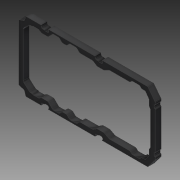
# Autodesk Inventor part: A0008269480
Saved by Autodesk Inventor 2014 SP2 (Build 180246200, 246)
## iProperties
Created: 2014-09-20
Part Number: A0008269480
Material: Rubber
Document SubType Name: Modeling
Designer: Lukasz Szmit
Density: 0.93 g/cm^3
Appearance: Rubber - Black - Version 1.1
Author: Lukasz Szmit
Autodesk Inventor part; units mm, degrees
ref_plane "YZ Plane" through (0, 0, 0) normal (1, 0, 0) x (0, 1, 0)
ref_plane "XZ Plane" through (0, 0, 0) normal (0, 1, 0) x (-1, 0, 0)
ref_plane "XY Plane" through (0, 0, 0) normal (0, 0, 1) x (1, 0, 0)
sketch "Sketch1" plane through (0, 0, 0) normal (0, 1, 0) x (-1, 0, 0)
  line L0 (206.8069, 83.1723) -> (206.8069, -83.1723)
  line L1 (193.4069, -67.3858) -> (193.4069, 67.3858)
  line L2 (-189.8501, 49.189) -> (-189.8501, -94.3805)
  line L3 (-189.4414, -50.7006) -> (-186.55, -55.6572)
  line L4 (-186.1413, -57.1689) -> (-186.1413, -72.6556)
  line L5 (-185.5922, -74.3857) -> (-175.4668, -88.73)
  line L6 (-200.9413, -60) -> (-200.9413, -64.9002)
  line L7 (-204.4413, -74.3803) -> (-204.4413, -69.2877)
  line L8 (-204.4501, -55.6105) -> (-204.4501, 55.6105)
  arc A0 (-203.2747, -67.8252) -> (-200.9413, -64.9002) centre (-203.9413, -64.9002) ccw
  arc A1 (-200.9413, -60) -> (-203.2805, -57.0737) centre (-203.9413, -60) ccw
  line L9 (-203.8197, -76.2088) -> (-182.8943, -103.4284)
  arc A2 (-182.8943, -103.4284) -> (-180.5159, -104.6) centre (-180.5159, -101.6) ccw
  arc A3 (-175.4668, -88.73) -> (-173.0159, -90) centre (-173.0159, -87) ccw
  arc A4 (-204.4413, -74.3803) -> (-203.8197, -76.2088) centre (-201.4413, -74.3803) ccw
  arc A5 (-186.1413, -72.6556) -> (-185.5922, -74.3857) centre (-183.1413, -72.6556) ccw
  arc A6 (-186.1413, -57.1689) -> (-186.55, -55.6572) centre (-189.1413, -57.1689) ccw
  arc A7 (-189.8501, -49.189) -> (-189.4414, -50.7006) centre (-186.8501, -49.189) ccw
  arc A8 (-204.4501, -55.6105) -> (-203.2805, -57.0737) centre (-202.9501, -55.6105) ccw
  arc A9 (-203.2747, -67.8252) -> (-204.4413, -69.2877) centre (-202.9413, -69.2877) ccw
  line L10 (-155.0159, -96.0718) -> (-137.0159, -96.0718)
  line L11 (-173.0159, -90) -> (-166.0159, -90)
  arc A10 (-126.0159, -90) -> (-131.5159, -93.0359) centre (-126.0159, -96.5) ccw
  arc A11 (-137.0159, -96.0718) -> (-131.5159, -93.0359) centre (-137.0159, -89.5718) ccw
  arc A12 (-160.5159, -93.0359) -> (-155.0159, -96.0718) centre (-155.0159, -89.5718) ccw
  arc A13 (-160.5159, -93.0359) -> (-166.0159, -90) centre (-166.0159, -96.5) ccw
  line L12 (-64.4945, -89.2551) -> (-51.3322, -82.3449)
  line L13 (-126.0159, -90) -> (-67.5159, -90)
  line L14 (-48.3108, -81.6) -> (-31.3108, -81.6)
  line L15 (-17.9251, -88.9697) -> (-27.7991, -82.6303)
  arc A14 (-67.5159, -90) -> (-64.4945, -89.2551) centre (-67.5159, -83.5) ccw
  arc A15 (-48.3108, -81.6) -> (-51.3322, -82.3449) centre (-48.3108, -88.1) ccw
  arc A16 (-17.9251, -88.9697) -> (-14.4134, -90) centre (-14.4134, -83.5) ccw
  arc A17 (-27.7991, -82.6303) -> (-31.3108, -81.6) centre (-31.3108, -88.1) ccw
  line L16 (-14.4134, -90) -> (20.5866, -90)
  line L17 (50.4322, -99.4607) -> (35.4322, -99.4607)
  line L18 (25.1828, -91.9038) -> (30.836, -97.5569)
  line L19 (60.6815, -91.9038) -> (55.0284, -97.5569)
  line L20 (65.2777, -90) -> (73.2777, -90)
  line L21 (77.8739, -91.9038) -> (83.527, -97.5569)
  arc A18 (25.1828, -91.9038) -> (20.5866, -90) centre (20.5866, -96.5) ccw
  arc A19 (50.4322, -99.4607) -> (55.0284, -97.5569) centre (50.4322, -92.9607) ccw
  arc A20 (65.2777, -90) -> (60.6815, -91.9038) centre (65.2777, -96.5) ccw
  arc A21 (77.8739, -91.9038) -> (73.2777, -90) centre (73.2777, -96.5) ccw
  arc A22 (30.836, -97.5569) -> (35.4322, -99.4607) centre (35.4322, -92.9607) ccw
  line L22 (88.1232, -99.4607) -> (101.1232, -99.4607)
  arc A23 (83.527, -97.5569) -> (88.1232, -99.4607) centre (88.1232, -92.9607) ccw
  line L23 (105.7194, -97.5569) -> (116.7725, -86.5038)
  arc A24 (101.1232, -99.4607) -> (105.7194, -97.5569) centre (101.1232, -92.9607) ccw
  line L24 (121.3687, -84.6) -> (136.3687, -84.6)
  line L25 (139.6187, -85.4708) -> (145.9551, -89.1292)
  arc A25 (121.3687, -84.6) -> (116.7725, -86.5038) centre (121.3687, -91.1) ccw
  arc A26 (139.6187, -85.4708) -> (136.3687, -84.6) centre (136.3687, -91.1) ccw
  arc A27 (145.9551, -89.1292) -> (149.2051, -90) centre (149.2051, -83.5) ccw
  line L26 (149.2051, -90) -> (163.3581, -90)
  line L27 (165.0901, -89) -> (164.9354, -89.2679)
  line L28 (166.4987, -88.2751) -> (171.369, -87.8626)
  line L29 (175.0876, -86.2889) -> (191.1741, -72.2889)
  arc A28 (163.3581, -90) -> (165.0901, -89) centre (163.3581, -88) ccw
  arc A29 (166.4987, -88.2751) -> (164.9354, -89.2679) centre (166.6675, -90.2679) ccw
  arc A30 (171.369, -87.8626) -> (175.0876, -86.2889) centre (170.8204, -81.3858) ccw
  arc A31 (191.1741, -72.2889) -> (193.4069, -67.3858) centre (186.9069, -67.3858) ccw
  line L30 (188.8967, -93.6379) -> (186.5552, -102.3765)
  line L31 (193.4929, -89.0417) -> (204.5834, -86.07)
  arc A32 (193.4929, -89.0417) -> (188.8967, -93.6379) centre (195.1753, -95.3202) ccw
  arc A33 (204.5834, -86.07) -> (206.8069, -83.1723) centre (203.8069, -83.1723) ccw
  arc A34 (183.6575, -104.6) -> (186.5552, -102.3765) centre (183.6575, -101.6) ccw
  line L32 (-41.4608, -99.75) -> (-36.5608, -99.75) construction
  line L33 (-36.5608, -94.9) -> (-41.4608, -94.9)
  arc A35 (-41.4608, -94.9) -> (-44.2842, -103.6935) centre (-41.4608, -99.75) ccw
  arc A36 (-32.7112, -96.8) -> (-36.5608, -94.9) centre (-36.5608, -99.75) ccw
  line L34 (-32.7112, -96.8) -> (-27.8608, -96.8)
  arc A37 (-23.0293, -101.2273) -> (-27.8608, -96.8) centre (-27.8608, -101.65) ccw
  line L35 (-44.5753, -104.6) -> (-180.5159, -104.6)
  line L36 (-22.7342, -104.6) -> (-23.0293, -101.2273)
  arc A38 (-44.5753, -104.6) -> (-44.2842, -103.6935) centre (-44.5753, -104.1) ccw
  line L37 (183.6575, -104.6) -> (139.6187, -104.6)
  line L38 (117.7776, -104.6) -> (-22.7342, -104.6)
  line L39 (-189.4414, 50.7006) -> (-186.55, 55.6572)
  line L40 (-186.1413, 57.1689) -> (-186.1413, 72.6556)
  line L41 (-185.5922, 74.3857) -> (-175.4668, 88.73)
  line L42 (-200.9413, 60) -> (-200.9413, 64.9002)
  line L43 (-204.4413, 74.3803) -> (-204.4413, 69.2877)
  arc A39 (-200.9413, 64.9002) -> (-203.2747, 67.8252) centre (-203.9413, 64.9002) ccw
  arc A40 (-203.2805, 57.0737) -> (-200.9413, 60) centre (-203.9413, 60) ccw
  line L44 (-203.8197, 76.2088) -> (-182.8943, 103.4284)
  arc A41 (-180.5159, 104.6) -> (-182.8943, 103.4284) centre (-180.5159, 101.6) ccw
  arc A42 (-173.0159, 90) -> (-175.4668, 88.73) centre (-173.0159, 87) ccw
  arc A43 (-203.8197, 76.2088) -> (-204.4413, 74.3803) centre (-201.4413, 74.3803) ccw
  arc A44 (-185.5922, 74.3857) -> (-186.1413, 72.6556) centre (-183.1413, 72.6556) ccw
  arc A45 (-186.55, 55.6572) -> (-186.1413, 57.1689) centre (-189.1413, 57.1689) ccw
  arc A46 (-189.4414, 50.7006) -> (-189.8501, 49.189) centre (-186.8501, 49.189) ccw
  arc A47 (-203.2805, 57.0737) -> (-204.4501, 55.6105) centre (-202.9501, 55.6105) ccw
  arc A48 (-204.4413, 69.2877) -> (-203.2747, 67.8252) centre (-202.9413, 69.2877) ccw
  line L45 (-155.0159, 96.0718) -> (-137.0159, 96.0718)
  line L46 (-173.0159, 90) -> (-166.0159, 90)
  arc A49 (-131.5159, 93.0359) -> (-126.0159, 90) centre (-126.0159, 96.5) ccw
  arc A50 (-131.5159, 93.0359) -> (-137.0159, 96.0718) centre (-137.0159, 89.5718) ccw
  arc A51 (-155.0159, 96.0718) -> (-160.5159, 93.0359) centre (-155.0159, 89.5718) ccw
  arc A52 (-166.0159, 90) -> (-160.5159, 93.0359) centre (-166.0159, 96.5) ccw
  line L47 (-64.4945, 89.2551) -> (-51.3322, 82.3449)
  line L48 (-126.0159, 90) -> (-67.5159, 90)
  line L49 (-48.3108, 81.6) -> (-31.3108, 81.6)
  line L50 (-17.9251, 88.9697) -> (-27.7991, 82.6303)
  arc A53 (-64.4945, 89.2551) -> (-67.5159, 90) centre (-67.5159, 83.5) ccw
  arc A54 (-51.3322, 82.3449) -> (-48.3108, 81.6) centre (-48.3108, 88.1) ccw
  arc A55 (-14.4134, 90) -> (-17.9251, 88.9697) centre (-14.4134, 83.5) ccw
  arc A56 (-31.3108, 81.6) -> (-27.7991, 82.6303) centre (-31.3108, 88.1) ccw
  line L51 (-14.4134, 90) -> (20.5866, 90)
  line L52 (50.4322, 99.4607) -> (35.4322, 99.4607)
  line L53 (25.1828, 91.9038) -> (30.836, 97.5569)
  line L54 (60.6815, 91.9038) -> (55.0284, 97.5569)
  line L55 (65.2777, 90) -> (73.2777, 90)
  line L56 (77.8739, 91.9038) -> (83.527, 97.5569)
  arc A57 (20.5866, 90) -> (25.1828, 91.9038) centre (20.5866, 96.5) ccw
  arc A58 (55.0284, 97.5569) -> (50.4322, 99.4607) centre (50.4322, 92.9607) ccw
  arc A59 (60.6815, 91.9038) -> (65.2777, 90) centre (65.2777, 96.5) ccw
  arc A60 (73.2777, 90) -> (77.8739, 91.9038) centre (73.2777, 96.5) ccw
  arc A61 (35.4322, 99.4607) -> (30.836, 97.5569) centre (35.4322, 92.9607) ccw
  line L57 (88.1232, 99.4607) -> (101.1232, 99.4607)
  arc A62 (88.1232, 99.4607) -> (83.527, 97.5569) centre (88.1232, 92.9607) ccw
  line L58 (105.7194, 97.5569) -> (116.7725, 86.5038)
  arc A63 (105.7194, 97.5569) -> (101.1232, 99.4607) centre (101.1232, 92.9607) ccw
  line L59 (121.3687, 84.6) -> (136.3687, 84.6)
  line L60 (139.6187, 85.4708) -> (145.9551, 89.1292)
  arc A64 (116.7725, 86.5038) -> (121.3687, 84.6) centre (121.3687, 91.1) ccw
  arc A65 (136.3687, 84.6) -> (139.6187, 85.4708) centre (136.3687, 91.1) ccw
  arc A66 (149.2051, 90) -> (145.9551, 89.1292) centre (149.2051, 83.5) ccw
  line L61 (149.2051, 90) -> (163.3581, 90)
  line L62 (165.0901, 89) -> (164.9354, 89.2679)
  line L63 (166.4987, 88.2751) -> (171.369, 87.8626)
  line L64 (175.0876, 86.2889) -> (191.1741, 72.2889)
  arc A67 (165.0901, 89) -> (163.3581, 90) centre (163.3581, 88) ccw
  arc A68 (164.9354, 89.2679) -> (166.4987, 88.2751) centre (166.6675, 90.2679) ccw
  arc A69 (175.0876, 86.2889) -> (171.369, 87.8626) centre (170.8204, 81.3858) ccw
  arc A70 (193.4069, 67.3858) -> (191.1741, 72.2889) centre (186.9069, 67.3858) ccw
  line L65 (188.8967, 93.6379) -> (186.5552, 102.3765)
  line L66 (193.4929, 89.0417) -> (204.5834, 86.07)
  arc A71 (188.8967, 93.6379) -> (193.4929, 89.0417) centre (195.1753, 95.3202) ccw
  arc A72 (206.8069, 83.1723) -> (204.5834, 86.07) centre (203.8069, 83.1723) ccw
  arc A73 (186.5552, 102.3765) -> (183.6575, 104.6) centre (183.6575, 101.6) ccw
  line L67 (-41.4608, 99.75) -> (-36.5608, 99.75) construction
  line L68 (-36.5608, 94.9) -> (-41.4608, 94.9)
  arc A74 (-44.2842, 103.6935) -> (-41.4608, 94.9) centre (-41.4608, 99.75) ccw
  arc A75 (-36.5608, 94.9) -> (-32.7112, 96.8) centre (-36.5608, 99.75) ccw
  line L69 (-32.7112, 96.8) -> (-27.8608, 96.8)
  arc A76 (-27.8608, 96.8) -> (-23.0293, 101.2273) centre (-27.8608, 101.65) ccw
  line L70 (-44.5753, 104.6) -> (-180.5159, 104.6)
  line L71 (-22.7342, 104.6) -> (-23.0293, 101.2273)
  arc A77 (-44.2842, 103.6935) -> (-44.5753, 104.6) centre (-44.5753, 104.1) ccw
  line L72 (183.6575, 104.6) -> (139.6187, 104.6)
  line L73 (117.7776, 104.6) -> (-22.7342, 104.6)
  line L74 (120.8921, 99.75) -> (125.7921, 99.75) construction
  line L75 (129.6418, 96.8) -> (134.4921, 96.8)
  line L76 (139.6187, 104.6) -> (139.3237, 101.2273)
  arc A78 (118.0687, 103.6935) -> (117.7776, 104.6) centre (117.7776, 104.1) ccw
  arc A79 (134.4921, 96.8) -> (139.3237, 101.2273) centre (134.4921, 101.65) ccw
  arc A80 (125.7921, 94.9) -> (129.6418, 96.8) centre (125.7921, 99.75) ccw
  line L77 (125.7921, 94.9) -> (120.8921, 94.9)
  arc A81 (118.0687, 103.6935) -> (120.8921, 94.9) centre (120.8921, 99.75) ccw
  arc A82 (117.7776, -104.6) -> (118.0687, -103.6935) centre (117.7776, -104.1) ccw
  arc A83 (120.8921, -94.9) -> (118.0687, -103.6935) centre (120.8921, -99.75) ccw
  line L78 (125.7921, -94.9) -> (120.8921, -94.9)
  line L79 (120.8921, -99.75) -> (125.7921, -99.75) construction
  line L80 (129.6418, -96.8) -> (134.4921, -96.8)
  arc A84 (139.3237, -101.2273) -> (134.4921, -96.8) centre (134.4921, -101.65) ccw
  line L81 (139.6187, -104.6) -> (139.3237, -101.2273)
  arc A85 (129.6418, -96.8) -> (125.7921, -94.9) centre (125.7921, -99.75) ccw
  point P0 (0, 0)
  point P1 (-204.4413, -75.4002)
  point P2 (-189.8501, -50)
  point P3 (-186.1413, -56.3578)
  point P4 (-186.1413, -73.6078)
  point P5 (-174.5704, -90)
  point P6 (-181.9937, -104.6)
  point P7 (-130.1639, -90)
  point P8 (-133.8735, -96)
  point P9 (-159.339, -96)
  point P10 (-162.3467, -90)
  point P11 (53.1245, -99.4607)
  point P12 (32.7398, -99.4607)
  point P13 (62.5853, -90)
  point P14 (70.5853, -90)
  point P15 (103.8156, -99.4607)
  point P16 (-204.4413, 75.4002)
  point P17 (-189.8501, 50)
  point P18 (-186.1413, 56.3578)
  point P19 (-186.1413, 73.6078)
  point P20 (-174.5704, 90)
  point P21 (-181.9937, 104.6)
  point P22 (-130.1639, 90)
  point P23 (-133.8735, 96)
  point P24 (-159.339, 96)
  point P25 (-162.3467, 90)
  point P26 (53.1245, 99.4607)
  point P27 (32.7398, 99.4607)
  point P28 (62.5853, 90)
  point P29 (70.5853, 90)
  point P30 (103.8156, 99.4607)
  point P31 (139.6187, -104.6)
  point P32 (117.7776, -104.6)
  dimension "d51" = 3
  dimension "d52" = 3
  dimension "d55" = 149.744
  dimension "d56" = 149.744
  dimension "d57" = 144.782
  dimension "d60" = 18.3
  dimension "d73" = 17.25
  dimension "d76" = 142.448
  dimension "d77" = 3
  dimension "d78" = 1.5
  dimension "d80" = 6.5
  dimension "d85" = 40
  dimension "d86" = 18
  dimension "d88" = 7
  dimension "d89" = 7.5
  dimension "d90" = 6.5
  dimension "d91" = 6.5
  dimension "d109" = 6.5
  dimension "d111" = 6.5
  dimension "d112" = 6.5
  dimension "d113" = 6.5
  dimension "d116" = 15
  dimension "d117" = 8
  dimension "d118" = 6.5
  dimension "d119" = 13
  dimension "d120" = 17
  dimension "d122" = 6.5
  dimension "d123" = 15
  dimension "d127" = 13.4
  dimension "d129" = 6.5
  dimension "d130" = 14
  dimension "d138" = 6.5
  dimension "d139" = 105
  dimension "d141" = 20
  dimension "d144" = 2
  dimension "d146" = 35
  dimension "d147" = 58.5
  dimension "d148" = 3
  dimension "d151" = 14.6
  dimension "d159" = 4.85
  dimension "d160" = 6.85
  dimension "d161" = 4.85
  dimension "d166" = 0.5
  dimension "d167" = 14.6
  dimension "d168" = 13.6
  dimension "d191" = 0.5
  dimension "d192" = 4.85
  dimension "d193" = 4.85
  dimension "d194" = 4.85
  dimension "d195" = 4.9
  dimension "d196" = 4.8503
  dimension "d197" = 95
  constraints: 172 end point, 172 point on circle, 86 centre point, 77 tangent, 39 point on line, 18 equal radius, 9 perpendicular, 2 coincident, 2 parallel
  measures "d51" radius of A0
  measures "d52" radius of A1
  measures "d55" angle of L3 L2
  measures "d56" angle of L4 L3
  measures "d57" angle of L5 L4
  measures "d60" horizontal distance of point (-204.441, -75.4) point (-186.141, -73.608)
  measures "d73" distance of point (-186.141, -56.358) point (-186.141, -73.608)
  measures "d76" angle of L9 L7
  measures "d77" radius of A2
  measures "d78" radius of A8
  measures "d80" radius of A10
  measures "d85" distance of A10.centre A13.centre
  measures "d86" distance of L10.start L10.end
  measures "d88" horizontal distance of A13.centre A3.centre
  measures "d89" horizontal distance of A3.centre A2.centre
  measures "d90" radius of A14
  measures "d91" radius of A17
  measures "d109" radius of A18
  measures "d111" radius of A20
  measures "d112" radius of A22
  measures "d113" radius of A23
  measures "d116" distance of A22.centre A19.centre
  measures "d117" distance of A20.centre A21.centre
  measures "d118" radius of A24
  measures "d119" distance of A23.centre A24.centre
  measures "d120" distance of A15.centre A17.centre
  measures "d122" radius of A25
  measures "d123" distance of A25.centre A26.centre
  measures "d127" distance between parallel lines of L0 L1
  measures "d129" radius of A30
  measures "d130" vertical distance of A31.centre A30.centre
  measures "d138" radius of A32
  measures "d139" angle of L0 L31
  measures "d141" distance from line of L29 A32.centre
  measures "d144" radius of A28
  measures "d146" horizontal distance of A18.centre A16.centre
  measures "d147" horizontal distance of A14.centre A10.centre
  measures "d148" radius of A34
  measures "d159" radius of A37
  measures "d160" horizontal distance of A15.centre L32.start
  measures "d161" radius of A35
  measures "d166" radius of A38
  measures "d167" distance between parallel lines of L8 L2
  measures "d168" horizontal distance of A37.centre L32.start
  measures "d191" radius of A82
  measures "d192" radius of A84
  measures "d193" radius of A85
  measures "d194" radius of A83
  measures "d195" distance of L78.start L78.end
  measures "d196" distance of L80.start L80.end
  measures "d197" angle of L37 L81
extrude "Extrusion2" add sketch "Sketch1" against normal blind 17.8
body "Solid2"
